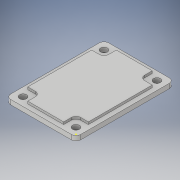
# Autodesk Inventor part: Tampa
Saved by Autodesk Inventor 2019 (Build 230136000, 136)
## iProperties
Created: 2021-05-27
Part Number: Tampa
Material: Generic
Document SubType Name: Modeling
Designer: hoope
Density: 1 g/cm^3
Appearance: Default
Author: hoope
Autodesk Inventor part; units mm, degrees
ref_plane "YZ Plane" through (0, 0, 0) normal (1, 0, 0) x (0, 1, 0)
ref_plane "XZ Plane" through (0, 0, 0) normal (0, 1, 0) x (-1, 0, 0)
ref_plane "XY Plane" through (0, 0, 0) normal (0, 0, 1) x (1, 0, 0)
sketch "Esboço1" plane through (0, 0, 0) normal (0, 1, 0) x (-1, 0, 0)
  line L0 (0, 0) -> (30, 0)
  line L1 (30, 0) -> (30, -42)
  line L2 (30, -42) -> (0, -42)
  line L3 (0, -42) -> (0, 0)
  dimension "d0" = 30
  dimension "d1" = 42
  constraints: 8 end point, 2 parallel, 1 horizontal, 1 perpendicular
  measures "d0" distance of L1.end L2.end
  measures "d1" distance of L0.end L1.end
extrude "Extrusão1" add sketch "Esboço1" along normal blind 2
fillet "Arredondamento1" radius 2 4 edges at (0, 1, 0) (0, 1, -42) (-30, 1, 0) (-30, 1, -42)
sketch "Esboço2" plane through (0, 2, 0) normal (0, 1, 0) x (1, 0, 0)
  line L0 (-28, 0) -> (-2, 0) projected
  line L1 (-30, 40) -> (-30, 2) projected
  line L2 (0, 2) -> (0, 40) projected
  line L3 (-2, 42) -> (-28, 42) projected
  line L4 (-2.01, 34.69) -> (-5.3, 34.69)
  line L5 (-24.69, 34.7) -> (-27.99, 34.7)
  line L6 (-2.01, 7.31) -> (-5.3, 7.31)
  line L7 (-24.69, 7.3) -> (-27.99, 7.3)
  line L8 (-7.3, 2.01) -> (-7.3, 5.31)
  line L9 (-7.3, 36.69) -> (-7.3, 39.99)
  line L10 (-22.69, 2.01) -> (-22.69, 5.3)
  line L11 (-22.69, 36.7) -> (-22.69, 39.99)
  arc A0 (-5.3, 7.31) -> (-7.3, 5.31) centre (-5.3, 5.31) ccw
  arc A1 (-22.69, 5.3) -> (-24.69, 7.3) centre (-24.69, 5.3) ccw
  arc A2 (-24.69, 34.7) -> (-22.69, 36.7) centre (-24.69, 36.7) ccw
  arc A3 (-7.3, 36.69) -> (-5.3, 34.69) centre (-5.3, 36.69) ccw
  line L12 (-7.3, 39.99) -> (-22.69, 39.99)
  line L13 (-27.99, 34.7) -> (-27.99, 7.3)
  line L14 (-22.69, 2.01) -> (-7.3, 2.01)
  line L15 (-2.01, 7.31) -> (-2.01, 34.69)
  point P0 (0, 0)
  dimension "d9" = 2
  dimension "d10" = 2.01
  dimension "d11" = 2.01
  dimension "d12" = 2.01
  dimension "d13" = 2.01
  constraints: 24 end point, 8 point on circle, 8 tangent, 4 centre point, 4 horizontal, 4 perpendicular, 4 vertical, 3 equal radius
  measures "d9" radius of A0
  measures "d10" distance between parallel lines of L3 L12
  measures "d11" distance between parallel lines of L2 L15
  measures "d12" distance between parallel lines of L0 L14
  measures "d13" distance between parallel lines of L1 L13
extrude "Extrusão2" add sketch "Esboço2" along normal blind 1
sketch "Esboço3" plane through (0, 2, 0) normal (0, 1, 0) x (1, 0, 0)
  circle A0 centre (-3.65, 3.65) radius 1.5
  circle A1 centre (-26.35, 38.35) radius 1.5
  line L0 (-30, 40) -> (-30, 2) projected
  line L1 (-2, 42) -> (-28, 42) projected
  line L2 (-28, 0) -> (-2, 0) projected
  line L3 (0, 2) -> (0, 40) projected
  circle A2 centre (-26.35, 3.65) radius 1.5
  circle A3 centre (-3.65, 38.35) radius 1.5
  point P0 (0, 0)
  dimension "d16" = 3
  dimension "d17" = 3
  dimension "d18" = 3.65
  dimension "d19" = 3.65
  dimension "d20" = 3.65
  dimension "d21" = 3.65
  dimension "d22" = 3
  dimension "d23" = 3
  constraints: 4 centre point
  measures "d16" diameter of A0
  measures "d17" diameter of A1
  measures "d18" distance from line of L0 A1.centre
  measures "d19" distance from line of L1 A1.centre
  measures "d20" distance from line of L2 A0.centre
  measures "d21" distance from line of L3 A0.centre
  measures "d22" diameter of A2
  measures "d23" diameter of A3
extrude "Extrusão3" cut sketch "Esboço3" against normal blind 3
sketch "Esboço4" plane through (0, 3, 0) normal (0, 1, 0) x (1, 0, 0)
  point P0 (0, 0)
